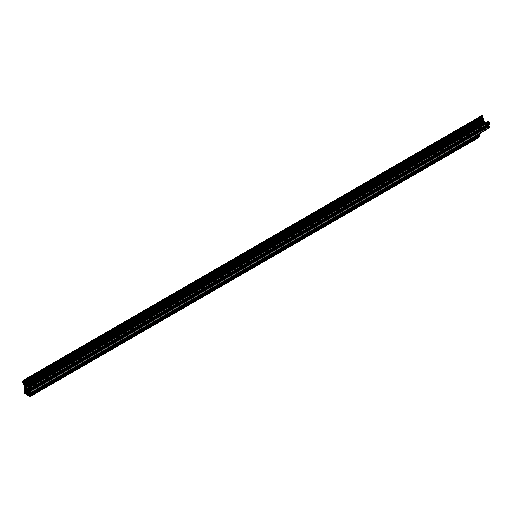
# Autodesk Inventor part: TL20240701-10100CV-DY1054-2-1
Saved by Autodesk Inventor 2022.5 (Build 265521000, 521)
## iProperties
Category: SUB ASSEMBLY NAME
Company: 현대 트랜시스
Created: 2023-04-05
Part Number: TL20240701-10100CV-DY1054-2-1
Checked By: 작성자
Engr Approved By: 윤수현
User Status: 2/2
Material: SS400
Description: 가공품
Document SubType Name: Modeling
Mfg Approved By: 호상태
Designer: 박성규
Stock Number: 부품 번호
Density: 7.85 g/cm^3
Appearance: 아노다이징 백색
Project: E.A PJT
DETAIL: Coveryor Assembly
M/C TITLE: CJ 제일제당 협동로봇 포장시스탬 PILOT 장비
PARTS NAME: Bracket
SPECIFICATION: TA20221101-CV200000-015
DocNumber: 221118_Standard_v1
Folder: .\
VDS_Category: 엔지니어링
Title: 도면 명
Subject: MEa차종 시트조립라인 3열 공정 개선 & 1열 방음실 설치
Author: 박성규
Revision Number: A
Autodesk Inventor part; units mm, degrees
ref_plane "YZ Plane" through (0, 0, 0) normal (1, 0, 0) x (0, 1, 0)
ref_plane "XZ Plane" through (0, 0, 0) normal (0, 1, 0) x (-1, 0, 0)
ref_plane "XY Plane" through (0, 0, 0) normal (0, 0, 1) x (1, 0, 0)
sketch "스케치9" plane through (0, 0, 0) normal (0, 0, 1) x (1, 0, 0)
  line L0 (40, 5.5) -> (35, 5.5)
  line L1 (35, 5.5) -> (35, 8)
  line L2 (35, 8) -> (29, 8)
  line L3 (29, 8) -> (29, 5.5)
  line L4 (29, 5.5) -> (27, 5.5)
  line L5 (27, 5.5) -> (27, -1.5)
  line L6 (29, -1.5) -> (29, -4)
  line L7 (29, -4) -> (35, -4)
  line L8 (35, -4) -> (35, -1.5)
  line L9 (35, -1.5) -> (40, -1.5)
  line L10 (40, -1.5) -> (40, -39.5)
  line L11 (40, -39.5) -> (35, -39.5)
  line L12 (35, -39.5) -> (35, -37)
  line L13 (35, -37) -> (29, -37)
  line L14 (29, -37) -> (29, -39.5)
  line L15 (29, -39.5) -> (18.5, -39.5)
  arc A0 (18.5, -39.5) -> (16.5, -41.5) centre (18.5, -41.5) ccw
  line L16 (16.5, -41.5) -> (16.5, -44.5)
  arc A1 (16.5, -44.5) -> (18.5, -46.5) centre (18.5, -44.5) ccw
  line L17 (18.5, -46.5) -> (29, -46.5)
  line L18 (29, -46.5) -> (29, -49)
  line L19 (29, -49) -> (35, -49)
  line L20 (35, -49) -> (35, -46.5)
  line L21 (35, -46.5) -> (40, -46.5)
  line L22 (40, -46.5) -> (40, -68)
  line L23 (40, -68) -> (4.25, -68)
  line L24 (4.25, -68) -> (4.25, -63)
  line L25 (4.25, -63) -> (8, -63)
  line L26 (8, -63) -> (8, -57)
  line L27 (8, -57) -> (4.25, -57)
  line L28 (4.25, -57) -> (4.25, -55)
  line L29 (4.25, -55) -> (-4.25, -55)
  line L30 (-4.25, -55) -> (-4.25, -57)
  line L31 (-4.25, -57) -> (-8, -57)
  line L32 (-8, -57) -> (-8, -63)
  line L33 (-8, -63) -> (-4.25, -63)
  line L34 (-4.25, -63) -> (-4.25, -68)
  line L35 (-4.25, -68) -> (-40, -68)
  line L36 (-40, -68) -> (-40, -46.5)
  line L37 (-40, -46.5) -> (-35, -46.5)
  line L38 (-35, -46.5) -> (-35, -49)
  line L39 (-35, -49) -> (-29, -49)
  line L40 (-29, -49) -> (-29, -46.5)
  line L41 (-29, -46.5) -> (-18.5, -46.5)
  arc A2 (-18.5, -46.5) -> (-16.5, -44.5) centre (-18.5, -44.5) ccw
  line L42 (-16.5, -44.5) -> (-16.5, -41.5)
  arc A3 (-16.5, -41.5) -> (-18.5, -39.5) centre (-18.5, -41.5) ccw
  line L43 (-18.5, -39.5) -> (-29, -39.5)
  line L44 (-29, -39.5) -> (-29, -37)
  line L45 (-29, -37) -> (-35, -37)
  line L46 (-35, -37) -> (-35, -39.5)
  line L47 (-35, -39.5) -> (-40, -39.5)
  line L48 (-40, -39.5) -> (-40, -1.5)
  line L49 (-40, -1.5) -> (-35, -1.5)
  line L50 (-35, -1.5) -> (-35, -4)
  line L51 (-35, -4) -> (-29, -4)
  line L52 (-29, -4) -> (-29, -1.5)
  line L53 (-29, -1.5) -> (-27, -1.5)
  line L54 (-27, -1.5) -> (-27, 5.5)
  line L55 (-27, 5.5) -> (-29, 5.5)
  line L56 (-29, 5.5) -> (-29, 8)
  line L57 (-29, 8) -> (-35, 8)
  line L58 (-35, 8) -> (-35, 5.5)
  line L59 (-35, 5.5) -> (-40, 5.5)
  line L60 (-40, 5.5) -> (-40, 22)
  line L61 (-40, 22) -> (-54, 38.6846)
  line L62 (-54, 38.6846) -> (-54, 65)
  arc A4 (-51, 68) -> (-54, 65) centre (-51, 65) ccw
  line L63 (-51, 68) -> (-40, 68)
  line L64 (-40, 68) -> (-40, 63.5)
  line L65 (-40, 63.5) -> (-43, 63.5)
  line L66 (-43, 63.5) -> (-43, 66)
  line L67 (-43, 66) -> (-49, 66)
  line L68 (-49, 66) -> (-49, 63.5)
  line L69 (27, -1.5) -> (29, -1.5)
  line L70 (-51.5, 63.5) -> (-51.5, 56.5)
  line L71 (-51.5, 56.5) -> (-49, 56.5)
  line L72 (-49, 56.5) -> (-49, 54)
  line L73 (-49, 54) -> (-43, 54)
  line L74 (-43, 54) -> (-43, 56.5)
  line L75 (-43, 56.5) -> (-40, 56.5)
  line L76 (-40, 56.5) -> (-40, 52)
  line L77 (-40, 52) -> (-45, 52)
  arc A5 (-45, 52) -> (-48, 49) centre (-45, 49) ccw
  line L78 (-48, 49) -> (-48, 43)
  arc A6 (-48, 43) -> (-45, 40) centre (-45, 43) ccw
  line L79 (-45, 40) -> (-38, 40)
  line L80 (-38, 40) -> (-38, 41)
  line L81 (-38, 41) -> (-34.5, 41)
  line L82 (-34.5, 41) -> (-34, 40)
  line L83 (-34, 40) -> (-33.5, 41)
  line L84 (-33.5, 41) -> (-30, 41)
  line L85 (-30, 41) -> (-30, 37)
  arc A7 (-32, 35) -> (-30, 37) centre (-32, 37) ccw
  line L86 (-32, 35) -> (-36, 35)
  line L87 (-36, 35) -> (-36, 20)
  arc A8 (-36, 20) -> (-31, 15) centre (-31, 20) ccw
  line L88 (-31, 15) -> (-25, 15)
  line L89 (-25, 15) -> (-25, 10.9)
  line L90 (-25, 10.9) -> (-17.5, 10.9)
  line L91 (-17.5, 10.9) -> (-17, 9.9)
  line L92 (-17, 9.9) -> (-16.5, 10.9)
  line L93 (-16.5, 10.9) -> (-9, 10.9)
  line L94 (-9, 10.9) -> (-9, 9.2)
  line L95 (-9, 9.2) -> (9, 9.2)
  line L96 (9, 9.2) -> (9, 10.9)
  line L97 (9, 10.9) -> (16.5, 10.9)
  line L98 (16.5, 10.9) -> (17, 9.9)
  line L99 (17, 9.9) -> (17.5, 10.9)
  line L100 (17.5, 10.9) -> (25, 10.9)
  line L101 (25, 10.9) -> (25, 15)
  line L102 (25, 15) -> (31, 15)
  arc A9 (31, 15) -> (36, 20) centre (31, 20) ccw
  line L103 (36, 20) -> (36, 35)
  line L104 (36, 35) -> (32, 35)
  arc A10 (30, 37) -> (32, 35) centre (32, 37) ccw
  line L105 (30, 37) -> (30, 41)
  line L106 (30, 41) -> (33.5, 41)
  line L107 (33.5, 41) -> (34, 40)
  line L108 (34, 40) -> (34.5, 41)
  line L109 (34.5, 41) -> (38, 41)
  line L110 (38, 41) -> (38, 40)
  line L111 (38, 40) -> (40, 40)
  line L112 (40, 40) -> (40, 5.5)
  line L113 (-23, 5) -> (23, 5)
  arc A11 (24, 4) -> (23, 5) centre (23, 4) ccw
  line L114 (24, 4) -> (24, -6)
  arc A12 (24, -6) -> (27, -9) centre (27, -6) ccw
  line L115 (27, -9) -> (34, -9)
  arc A13 (37, -12) -> (34, -9) centre (34, -12) ccw
  line L116 (37, -12) -> (37, -32)
  arc A14 (34, -35) -> (37, -32) centre (34, -32) ccw
  line L117 (34, -35) -> (9.25, -35)
  line L118 (9.25, -35) -> (9.25, -39.5)
  line L119 (9.25, -39.5) -> (12.75, -39.5)
  line L120 (12.75, -39.5) -> (12.75, -50)
  line L121 (12.75, -50) -> (-12.75, -50)
  line L122 (-12.75, -50) -> (-12.75, -39.5)
  line L123 (-12.75, -39.5) -> (-9.25, -39.5)
  line L124 (-9.25, -39.5) -> (-9.25, -35)
  line L125 (-9.25, -35) -> (-34, -35)
  arc A15 (-37, -32) -> (-34, -35) centre (-34, -32) ccw
  line L126 (-49, 63.5) -> (-51.5, 63.5)
  arc A16 (-34, -9) -> (-37, -12) centre (-34, -12) ccw
  line L127 (-34, -9) -> (-27, -9)
  arc A17 (-27, -9) -> (-24, -6) centre (-27, -6) ccw
  line L128 (-24, -6) -> (-24, 4)
  arc A18 (-23, 5) -> (-24, 4) centre (-23, 4) ccw
  arc A19 (37, -55) -> (34, -52) centre (34, -55) ccw
  line L129 (34, -52) -> (14, -52)
  arc A20 (14, -52) -> (11, -55) centre (14, -55) ccw
  line L130 (11, -55) -> (11, -62)
  arc A21 (11, -62) -> (14, -65) centre (14, -62) ccw
  line L131 (14, -65) -> (34, -65)
  arc A22 (34, -65) -> (37, -62) centre (34, -62) ccw
  line L132 (37, -62) -> (37, -55)
  arc A23 (-37, -62) -> (-34, -65) centre (-34, -62) ccw
  line L133 (-34, -65) -> (-14, -65)
  arc A24 (-14, -65) -> (-11, -62) centre (-14, -62) ccw
  line L134 (-11, -62) -> (-11, -55)
  arc A25 (-11, -55) -> (-14, -52) centre (-14, -55) ccw
  line L135 (-14, -52) -> (-34, -52)
  arc A26 (-34, -52) -> (-37, -55) centre (-34, -55) ccw
  line L136 (-37, -55) -> (-37, -62)
  circle A27 centre (-42, 34) radius 4
  line L137 (-37, -32) -> (-37, -12)
  point P0 (0, 0)
  point P1 (0, 0)
  point P2 (-41.1372, 2)
  point P3 (-40.2674, -43)
  constraints: 276 end point, 54 point on circle, 28 centre point
extrude "돌출4" add sketch "스케치9" along normal mid plane 6000
sketch "스케치10" plane through (40, -46.5, 3000) normal (1, 0, 0) x (0, 0, -1)
  line L0 (6000, -21.5) -> (0, -21.5) construction
  line L1 (0, -21.5) -> (130, -21.5)
  line L2 (130, -21.5) -> (130, 18.5)
  line L3 (130, 18.5) -> (0, 18.5)
  line L4 (0, 18.5) -> (0, -21.5)
  line L5 (6000, -21.5) -> (5870, -21.5)
  line L6 (5870, -21.5) -> (5870, 18.5)
  line L7 (5870, 18.5) -> (6000, 18.5)
  line L8 (6000, 18.5) -> (6000, -21.5)
  point P0 (3000, 46.5)
  dimension "d42" = 40
  dimension "d43" = 130
  dimension "d44" = 130
  constraints: 16 end point, 4 parallel, 2 horizontal, 2 perpendicular, 1 point on line
  measures "d42" distance of L5.end L6.end
  measures "d43" distance of L6.end L7.end
  measures "d44" distance of L2.end L3.end
extrude "돌출5" cut sketch "스케치10" against normal through all contours L5 L6 L7 L8
equation "\"d40\" = L1"
equation "\"d44\" = d43"
equation "\"L1\" = 6000"
